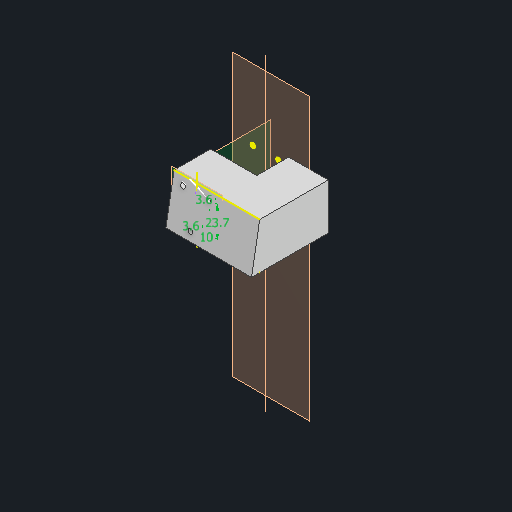
# Autodesk Inventor part: Camera_mount_angled
Saved by Autodesk Inventor 2027.1 (Build 311270010, 270A)
## iProperties
Created: 2026-09-16
Part Number: Camera_mount_angled
Material: Generic
Document SubType Name: Modeling
Designer: Jacob Parker
Density: 1 g/cm^3
Appearance: Default
Author: Jacob Parker
Autodesk Inventor part; units mm, degrees
ref_plane "YZ Plane" through (0, 0, 0) normal (1, 0, 0) x (0, 1, 0)
ref_plane "XZ Plane" through (0, 0, 0) normal (0, 1, 0) x (-1, 0, 0)
ref_plane "XY Plane" through (0, 0, 0) normal (0, 0, 1) x (1, 0, 0)
ref_plane "Work Plane1" through (4.4043, -35.2586, 0) normal (0, 0, 1) x (1, 0, 0)
ref_plane "Work Plane2" through (-18, 18, 0) normal (-1, 0, 0) x (0, -1, 0)
sketch "Sketch2" plane through (-18, 18, 0) normal (-1, 0, 0) x (0, -1, 0)
  line L0 (-7.4291, 0) -> (28.5709, 0)
  line L1 (28.5709, 0) -> (28.5709, 60)
  line L2 (-7.4291, 0) -> (-7.4291, 53.6522)
  line L3 (-7.4291, 53.6522) -> (28.5709, 60)
  point P0 (14.2854, 0)
  dimension "d7" = 60
  dimension "d56" = 36
  dimension "d59" = 80
  constraints: 8 end point, 2 vertical
  measures "d7" distance of L0.end L1.end
  measures "d56" distance of L0.start L0.end
  measures "d59" angle of L1 L3
extrude "Extrusion1" add sketch "Sketch2" against normal blind 67
ref_plane "Work Plane3" through (-18, 25.4291, 53.6522) normal (0, 0, -1) x (1, 0, 0)
sketch "Sketch3" plane through (-18, 25.4291, 53.6522) normal (0, 0, -1) x (1, 0, 0)
  line L0 (18, 43.2) -> (18, -7.2) projected
  circle A0 centre (18, 29.85) radius 1.8
  circle A1 centre (28, 6.15) radius 1.8
  circle A2 centre (8, 6.15) radius 1.8
  line L1 (18, 29.85) -> (33.5, 36)
  line L2 (0, 36) -> (67, 36) projected
  line L3 (28, 6.15) -> (12.5, 0)
  line L4 (0, 0) -> (67, 0) projected
  point P0 (18, 25.4291)
  point P1 (18, 6.0253)
  point P2 (29.4211, 27.8342)
  point P3 (6.5789, 27.8342)
  dimension "d33" = 3.6
  dimension "d34" = 3.6
  dimension "d57" = 23.7
  dimension "d58" = 10
  constraints: 4 end point, 3 centre point, 2 parallel, 2 point on line, 1 midpoint, 1 symmetric about line, 1 other
  measures "d33" diameter of A0
  measures "d34" diameter of A1
  measures "d57" vertical distance of L1.start L3.start
  measures "d58" horizontal distance of L3.start L1.start
hole "Hole4" at (10, 19.2791, 53.6522) at (0, -4.4209, 53.6522) at (-10, 19.2791, 53.6522) direction (0, 0, 1) diameter 3.6 end through all
hole "Hole5" at (10, 19.2791, 53.6522) at (-10, 19.2791, 53.6522) at (0, -4.4209, 53.6522) direction (0, 0, -1) diameter 3.6 end through all
sketch "Sketch5" plane through (-18, -10.5709, 0) normal (0, 0, -1) x (-1, 0, 0)
  circle A0 centre (-8, 29.85) radius 1.8 projected
  circle A1 centre (-18, 6.15) radius 1.8 projected
  circle A2 centre (-28, 29.85) radius 1.8 projected
  point P0 (-18, 10.5709)
hole "Hole6" at (-10, 19.2791, 0) at (10, 19.2791, 0) direction (0, 0, 1) diameter 6.5 depth 48.652
hole "Hole7" at (0, -4.4209, 0) direction (0, 0, 1) diameter 6.5 depth 55
sketch "Sketch6" plane through (-18, -10.5709, 0) normal (0, 0, -1) x (-1, 0, 0)
  line L0 (0, 0) -> (0, 36) projected
  line L1 (0, 0) -> (-36, 0)
  line L2 (-36, 0) -> (-36, 36)
  line L3 (-36, 36) -> (0, 36)
  line L4 (0, 36) -> (0, 0)
  point P0 (-18, 10.5709)
  dimension "d67" = 36
  dimension "d68" = 36
  constraints: 8 end point, 2 parallel, 1 horizontal, 1 perpendicular
  measures "d67" distance of L2.end L3.end
  measures "d68" distance of L1.end L2.end
extrude "Extrusion2" cut sketch "Sketch6" against normal blind 25
body "Solid1"
